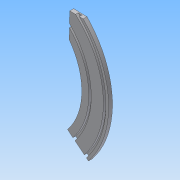
# Autodesk Inventor part: HOT Thermo bulb outline R
Saved by Autodesk Inventor 2013 (Build 170138000, 138)
## iProperties
Created: 2018-07-29
Part Number: HOT Thermo bulb outline R
Material: Generic
Document SubType Name: Modeling
Designer: Jeff Vyduna
Density: 1 g/cm^3
Author: Jeff Vyduna
Autodesk Inventor part; units mm, degrees
ref_plane "YZ Plane" through (0, 0, 0) normal (1, 0, 0) x (0, 1, 0)
ref_plane "XZ Plane" through (0, 0, 0) normal (0, 1, 0) x (-1, 0, 0)
ref_plane "XY Plane" through (0, 0, 0) normal (0, 0, 1) x (1, 0, 0)
ref_plane "Work Plane1" through (22.5184, 2.463, -18.3509) normal (0, 0, 1) x (0.9997722, -0.0213418, 0)
sketch "ThermoBulbBorder" plane through (22.5184, 2.463, -18.3509) normal (0, 0, 1) x (0.9997722, -0.0213418, 0)
  arc A0 (-447.455, -468.958) -> (162.145, -468.958) centre (-142.655, -774.8145) ccw
  arc A1 (-447.455, -468.958) -> (162.145, -468.958) centre (-142.655, -774.8145) ccw
  arc A2 (-383.955, -588.5959) -> (98.645, -588.5959) centre (-142.655, -774.8145) ccw
  line L0 (-447.455, -468.958) -> (-383.955, -468.958)
  line L1 (-383.955, -468.958) -> (-383.955, -588.5959)
  line L2 (162.145, -468.958) -> (98.645, -468.958)
  line L3 (98.645, -468.958) -> (98.645, -588.5959)
  line L4 (-383.955, -961.033) -> (-484.4967, -1038.6241)
  line L5 (98.645, -961.033) -> (199.1867, -1038.6241)
  arc A3 (-447.455, -468.958) -> (162.145, -468.958) centre (-142.655, -774.8145) ccw projected
  circle A4 centre (-142.655, -774.8145) radius 419.1 construction
  circle A5 centre (-142.655, -774.8145) radius 410.972 construction
  circle A6 centre (-142.655, -774.8145) radius 353.822 construction
  circle A7 centre (-142.655, -774.8145) radius 345.694 construction
  line L6 (98.645, -468.958) -> (98.645, -316.558) construction
  line L7 (-383.955, -468.958) -> (-383.955, -316.558) construction
  dimension "d0" = 609.6
  dimension "d5" = 63.5
  dimension "d6" = 63.5
  dimension "d7" = 838.2
  dimension "d8" = 8.128
  dimension "d9" = 8.128
  dimension "d10" = 57.15
  dimension "d11" = 40.894
  dimension "d12" = 152.4
  constraints: 16 end point, 12 point on circle, 7 centre point, 5 coincident, 2 concentric, 2 horizontal, 2 horizontal alignment, 2 line through centre, 2 parallel, 2 vertical, 2 vertical alignment, 1 collinear
  measures "d0" diameter of A2
  measures "d5" distance of L0.start L0.end
  measures "d6" distance of L2.start L2.end
  measures "d7" diameter of A4
  measures "d8" radial gap between concentric circles of A4 A5
  measures "d9" radial gap between concentric circles of A7 A6
  measures "d10" radial gap between concentric circles of A5 A6
  measures "d11" radial gap between concentric circles of A7 A2
  measures "d12" distance of L2.end L6.end
extrude "Extrusion3" add sketch "ThermoBulbBorder" along normal blind 18.034 contours L5 A2 L3 L2 A0
sketch "Sketch2" plane through (22.5184, 2.463, -0.3169) normal (0, 0, 1) x (0.9997722, -0.0213418, 0)
  line L0 (149.445, -468.958) -> (137.253, -468.958)
  arc A0 (199.1867, -1038.6241) -> (162.145, -468.958) centre (-142.655, -774.8145) ccw projected
  arc A1 (124.5847, -981.0515) -> (98.645, -538.7528) centre (-142.655, -774.8145) ccw
  arc A2 (134.2367, -988.5003) -> (98.645, -521.6249) centre (-142.655, -774.8145) ccw
  arc A3 (179.4805, -1023.4163) -> (144.5742, -486.5897) centre (-142.655, -774.8145) ccw
  arc A4 (189.1325, -1030.865) -> (153.1803, -477.9538) centre (-142.655, -774.8145) ccw
  line L1 (162.145, -468.958) -> (98.645, -468.958) projected
  line L2 (98.645, -961.033) -> (199.1867, -1038.6241) projected
  line L3 (98.645, -538.7528) -> (98.645, -521.6249)
  line L4 (98.645, -468.958) -> (98.645, -588.5959) projected
  line L5 (124.5847, -981.0515) -> (134.2367, -988.5003)
  line L6 (179.4805, -1023.4163) -> (189.1325, -1030.865)
  line L7 (149.445, -468.958) -> (149.445, -443.558) construction
  arc A5 (149.445, -468.958) -> (153.1803, -477.9538) centre (162.145, -468.958) ccw
  line L8 (137.253, -468.958) -> (137.253, -443.558) construction
  arc A6 (137.253, -468.958) -> (144.5742, -486.5897) centre (162.145, -468.958) ccw
  point P0 (-22.4607, -2.943)
  dimension "d17" = 12.7
  dimension "bRopeChannel" = 12.192
  dimension "d19" = 12.192
  dimension "d20" = 57.15
  dimension "d23" = 12.7
  dimension "d24" = 25.4
  dimension "d25" = 12.192
  constraints: 12 end point, 12 point on circle, 6 centre point, 5 collinear, 4 concentric, 4 tangent, 3 point on line, 2 parallel, 1 horizontal alignment
  measures "d17" radial gap between concentric circles of A0 A4
  measures "bRopeChannel" radial gap between concentric circles of A4 A3
  measures "d19" radial gap between concentric circles of A1 A2
  measures "d20" radial gap between concentric circles of A3 A2
  measures "d23" distance of L0.start L1.start
  measures "d24" distance of L0.start L7.end
  measures "d25" distance between parallel lines of L8 L7
extrude "Extrusion4" cut sketch "Sketch2" against normal blind 12.7 contours A5 A4 L2 A3 A6 L0 | A2 L2 A1 L3
equation "\"d6\" = d5"
equation "\"d8\" = sRopeChannel"
equation "\"d9\" = sRopeChannel"
equation "\"d19\" = bRopeChannel"
equation "\"d23\" = d17"
equation "\"sRopeChannel\" = 8.128"
body "Solid2"
